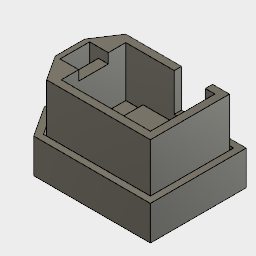
trrs-wssm-housing (Autodesk Fusion 360 design; units mm, degrees)
Autodesk Fusion 360 part; units mm, degrees
sketch "Sketch1" plane through (0, 0, 0) normal (0, 1, 0) x (1, 0, 0)
  line L0 (10.55, -8.05) -> (-10.55, -8.05)
  line L1 (-10.55, -8.05) -> (-10.55, 8.05)
  line L2 (-10.55, 8.05) -> (10.55, 8.05)
  line L3 (10.55, 8.05) -> (10.55, -8.05)
  line L4 (10.55, -8.05) -> (-10.55, 8.05) construction
  line L5 (-10.55, -8.05) -> (10.55, 8.05) construction
  dimension "d1" = 21.1
  dimension "d2" = 16.1
  measures "d1" distance of L1.end L2.end
  measures "d2" distance of L0.end L1.end
extrude "Extrude1" add sketch "Sketch1" along normal blind 3.5 makes body 1
sketch "Sketch2" plane through (0, 3.5, 0) normal (0, 1, 0) x (-1, 0, 0)
  line L0 (-10.55, -8.05) -> (10.55, -8.05)
  line L1 (10.55, -8.05) -> (10.55, 8.05)
  line L2 (10.55, 8.05) -> (-10.55, 8.05)
  line L3 (-10.55, 8.05) -> (-10.55, -8.05)
  line L4 (-9.05, 6.55) -> (9.05, 6.55)
  line L5 (9.05, 6.55) -> (9.05, -6.55)
  line L6 (9.05, -6.55) -> (-9.05, -6.55)
  line L7 (-9.05, -6.55) -> (-9.05, 6.55)
  line L8 (-9.05, 6.55) -> (9.05, -6.55) construction
  line L9 (9.05, 6.55) -> (-9.05, -6.55) construction
  dimension "d5" = 18.1
  dimension "d6" = 13.1
  measures "d5" distance of L5.end L6.end
  measures "d6" distance of L4.end L5.end
extrude "Extrude2" cut sketch "Sketch2" against normal blind 1.5 contours L4 L5 L6 L7 bodies 1
extrude "Extrude3" add 1 faces at (-3.0167, 3.5, -7.55) along direction (0, 1, 0) blind 5.7 on bodies 1 bodies 1
sketch "Sketch3" plane through (0, 9.2, 0) normal (0, 1, 0) x (-1, 0, 0)
  line L0 (9.05, 6.55) -> (9.05, -6.55)
  line L1 (9.05, -6.55) -> (-9.05, -6.55)
  line L2 (-9.05, -6.55) -> (-9.05, 6.55)
  line L3 (-9.05, 6.55) -> (9.05, 6.55)
  line L4 (-10.55, -8.05) -> (10.55, -8.05)
  line L5 (10.55, -8.05) -> (10.55, 8.05)
  line L6 (10.55, 8.05) -> (-10.55, 8.05)
  line L7 (-10.55, 8.05) -> (-10.55, -8.05)
  line L8 (-9.05, -6.55) -> (-7.1, -6.55)
  line L9 (-7.1, -6.55) -> (-7.1, -8.05)
  line L10 (-7.1, -8.05) -> (-9.05, -8.05)
  line L11 (-9.05, -8.05) -> (-9.05, -6.55)
  line L12 (-7.1, -6.55) -> (-0.8, -6.55)
  line L13 (-0.8, -6.55) -> (-0.8, -8.05)
  line L14 (-0.8, -8.05) -> (-7.1, -8.05)
  line L15 (-7.1, -8.05) -> (-7.1, -6.55)
  dimension "d11" = 1.95
  dimension "d12" = 6.3
  measures "d11" distance of L1.end L8.end
  measures "d12" distance of L8.end L12.end
extrude "Extrude4" cut sketch "Sketch3" against normal blind 5.7 contours L1 L4 L9 L12 L13 L14 L15 bodies 1
sketch "Sketch4" plane through (0, 2, 0) normal (0, 1, 0) x (-1, 0, 0)
  line L0 (-9.05, -6.55) -> (9.05, -6.55)
  line L1 (9.05, -6.55) -> (9.05, 6.55)
  line L2 (9.05, 6.55) -> (-9.05, 6.55)
  line L3 (-9.05, 6.55) -> (-9.05, -6.55)
  line L4 (-0.8, -6.55) -> (-7.1, -6.55)
  line L5 (-7.1, -6.55) -> (-7.1, -8.05)
  line L6 (-7.1, -8.05) -> (-0.8, -8.05)
  line L7 (-0.8, -8.05) -> (-0.8, -6.55)
  line L8 (9.05, -6.55) -> (5.55, -6.55)
  line L9 (5.55, -6.55) -> (5.55, 6.55)
  line L10 (5.55, 6.55) -> (9.05, 6.55)
  line L11 (9.05, 6.55) -> (9.05, -6.55)
  dimension "d15" = 3.5
  measures "d15" distance of L0.end L8.end
extrude "Extrude5" cut sketch "Sketch4" against normal blind 1 contours L0 L1 L2 L8 L9 L10 L11 bodies 1
sketch "Sketch5" plane through (0, 9.2, 0) normal (0, 1, 0) x (-1, 0, 0)
  line L0 (-7.1, -8.05) -> (-7.1, -6.55)
  line L1 (-7.1, -6.55) -> (-9.05, -6.55)
  line L2 (-9.05, -6.55) -> (-9.05, 6.55)
  line L3 (-9.05, 6.55) -> (9.05, 6.55)
  line L4 (9.05, 6.55) -> (9.05, -6.55)
  line L5 (9.05, -6.55) -> (-0.8, -6.55)
  line L6 (-0.8, -6.55) -> (-0.8, -8.05)
  line L7 (-0.8, -8.05) -> (10.55, -8.05)
  line L8 (10.55, -8.05) -> (10.55, 8.05)
  line L9 (10.55, 8.05) -> (-10.55, 8.05)
  line L10 (-10.55, 8.05) -> (-10.55, -8.05)
  line L11 (-10.55, -8.05) -> (-7.1, -8.05)
  line L12 (12.85, -3) -> (8.25, -3)
  line L13 (8.25, -3) -> (8.25, 3)
  line L14 (8.25, 3) -> (12.85, 3)
  line L15 (12.85, 3) -> (12.85, -3)
  line L16 (12.85, -3) -> (8.25, 3) construction
  line L17 (8.25, -3) -> (12.85, 3) construction
  line L18 (12.85, -3) -> (13.85, -3)
  line L19 (13.85, -3) -> (13.85, 3)
  line L20 (13.85, 3) -> (12.85, 3)
  line L21 (12.85, 3) -> (12.85, -3)
  line L22 (10.55, -8.05) -> (10.55, 8.05)
  line L23 (10.55, 8.05) -> (13.85, 3)
  line L24 (13.85, -3) -> (10.55, -8.05)
  point P0 (10.55, 0)
  dimension "d18" = 4.6
  dimension "d19" = 6
  dimension "d20" = 1
  measures "d18" distance of L13.end L14.end
  measures "d19" distance of L12.end L13.end
  measures "d20" distance of L12.start L18.end
extrude "Extrude6" add sketch "Sketch5" against normal blind 9.2 contours L8 L14 L20 L22 L23 | L8 L12 L14 L15 L21 L22 | L15 L18 L19 L20 L21 | L8 L12 L18 L22 L24 bodies 1
sketch "Sketch6" plane through (0, 9.2, 0) normal (0, 1, 0) x (-1, 0, 0)
  line L0 (-7.1, -8.05) -> (-7.1, -6.55)
  line L1 (-7.1, -6.55) -> (-9.05, -6.55)
  line L2 (-9.05, -6.55) -> (-9.05, 6.55)
  line L3 (-9.05, 6.55) -> (9.05, 6.55)
  line L4 (9.05, 6.55) -> (9.05, -6.55)
  line L5 (9.05, -6.55) -> (-0.8, -6.55)
  line L6 (-0.8, -6.55) -> (-0.8, -8.05)
  line L7 (-0.8, -8.05) -> (10.55, -8.05)
  line L8 (10.55, -8.05) -> (13.85, -3)
  line L9 (13.85, -3) -> (13.85, 3)
  line L10 (13.85, 3) -> (10.55, 8.05)
  line L11 (10.55, 8.05) -> (-10.55, 8.05)
  line L12 (-10.55, 8.05) -> (-10.55, -8.05)
  line L13 (-10.55, -8.05) -> (-7.1, -8.05)
  line L14 (13.85, -3) -> (12.85, -3)
  line L15 (12.85, -3) -> (12.85, 3)
  line L16 (12.85, 3) -> (13.85, 3)
  line L17 (13.85, 3) -> (13.85, -3)
  line L18 (12.85, -3) -> (11.05, -3)
  line L19 (11.05, -3) -> (11.05, 3)
  line L20 (11.05, 3) -> (12.85, 3)
  line L21 (12.85, 3) -> (12.85, -3)
  dimension "d23" = 1
  dimension "d24" = 1.8
  measures "d23" distance of L8.end L14.end
  measures "d24" distance of L14.end L18.end
extrude "Extrude7" cut sketch "Sketch6" against normal blind 7.2 contours L15 L18 L19 L20 L21 bodies 1
extrude "Extrude8" add 1 faces at (-9.7167, 9.2, -1) along direction (0, 1, 0) blind 2 on bodies 1 bodies 1
sketch "Sketch7" plane through (0, 11.2, 0) normal (0, 1, 0) x (-1, 0, 0)
  line L0 (11.05, -3) -> (11.05, 3)
  line L1 (11.05, 3) -> (12.85, 3)
  line L2 (12.85, 3) -> (12.85, -3)
  line L3 (12.85, -3) -> (11.05, -3)
  line L4 (-7.1, -8.05) -> (-7.1, -6.55)
  line L5 (-7.1, -6.55) -> (-9.05, -6.55)
  line L6 (-9.05, -6.55) -> (-9.05, 6.55)
  line L7 (-9.05, 6.55) -> (9.05, 6.55)
  line L8 (9.05, 6.55) -> (9.05, -6.55)
  line L9 (9.05, -6.55) -> (-0.8, -6.55)
  line L10 (-0.8, -6.55) -> (-0.8, -8.05)
  line L11 (-0.8, -8.05) -> (10.55, -8.05)
  line L12 (10.55, -8.05) -> (13.85, -3)
  line L13 (13.85, -3) -> (13.85, 3)
  line L14 (13.85, 3) -> (10.55, 8.05)
  line L15 (10.55, 8.05) -> (-10.55, 8.05)
  line L16 (-10.55, 8.05) -> (-10.55, -8.05)
  line L17 (-10.55, -8.05) -> (-7.1, -8.05)
  line L18 (11.05, -3) -> (9.05, -3)
  line L19 (9.05, -3) -> (9.05, 3)
  line L20 (9.05, 3) -> (11.05, 3)
  line L21 (11.05, 3) -> (11.05, -3)
extrude "Extrude9" cut sketch "Sketch7" against normal blind 2 contours L0 L8 L18 L19 L20 L21 bodies 1
copy_body "Body->Comp1" bodies 1 removing the originals makes body 2 in component "WSSM-03: Lower Half "
sketch "Sketch1 (2)" plane through (0, 11.2, 0) normal (0, 1, 0) x (-1, 0, 0) in component "WSSM-04: Upper Half"
  line L0 (9.05, 3) -> (12.85, 3)
  line L1 (12.85, 3) -> (12.85, -3)
  line L2 (12.85, -3) -> (9.05, -3)
  line L3 (9.05, -3) -> (9.05, -6.55)
  line L4 (9.05, -6.55) -> (-0.8, -6.55)
  line L5 (-0.8, -6.55) -> (-0.8, -8.05)
  line L6 (-0.8, -8.05) -> (10.55, -8.05)
  line L7 (10.55, -8.05) -> (13.85, -3)
  line L8 (13.85, -3) -> (13.85, 3)
  line L9 (13.85, 3) -> (10.55, 8.05)
  line L10 (10.55, 8.05) -> (-10.55, 8.05)
  line L11 (-10.55, 8.05) -> (-10.55, -8.05)
  line L12 (-10.55, -8.05) -> (-7.1, -8.05)
  line L13 (-7.1, -8.05) -> (-7.1, -6.55)
  line L14 (-7.1, -6.55) -> (-9.05, -6.55)
  line L15 (-9.05, -6.55) -> (-9.05, 6.55)
  line L16 (-9.05, 6.55) -> (9.05, 6.55)
  line L17 (9.05, 6.55) -> (9.05, 3)
  line L18 (-9.05, 6.55) -> (-0.8, 6.55)
  line L19 (-0.8, 6.55) -> (-0.8, -6.55)
  line L20 (-0.8, -6.55) -> (-9.05, -6.55)
  line L21 (-9.05, -6.55) -> (-9.05, 6.55)
  line L22 (-0.8, -8.05) -> (-7.1, -8.05)
  line L23 (-7.1, -8.05) -> (-7.1, -6.55)
  line L24 (-7.1, -6.55) -> (-0.8, -6.55)
  line L25 (-0.8, -6.55) -> (-0.8, -8.05)
extrude "Extrude1'" add sketch "Sketch1 (2)" against normal blind 1.85 separate body contours L14 L15 L16 L18 L19 L20 L21 L24 | L5 L13 L20 L22 L23 L24 L25 makes body 3 in component "WSSM-04: Upper Half"
move_face "OffsetFaces1" offset -0.09 1 faces at (9.05, 10.5833, -2.1833) on bodies 3 in component "WSSM-04: Upper Half"
move_face "OffsetFaces2" offset -0.09 1 faces at (3.52, 9.9667, 6.55) on bodies 3 in component "WSSM-04: Upper Half"
move_face "OffsetFaces3" offset -0.09 1 faces at (7.72, 10.5833, -6.55) on bodies 3 in component "WSSM-04: Upper Half"
move_face "OffsetFaces4" offset -0.15 1 faces at (7.1, 10.5833, -7.52) on bodies 3 in component "WSSM-04: Upper Half"
sketch "Sketch2 (2)" plane through (0, 11.2, 0) normal (0, 1, 0) x (-1, 0, 0) in component "WSSM-04: Upper Half"
  line L0 (9.05, 3) -> (12.85, 3)
  line L1 (12.85, 3) -> (12.85, -3)
  line L2 (12.85, -3) -> (9.05, -3)
  line L3 (9.05, -3) -> (9.05, -6.55)
  line L4 (9.05, -6.55) -> (-0.8, -6.55)
  line L5 (-0.8, -6.55) -> (-0.8, -8.05)
  line L6 (-0.8, -8.05) -> (10.55, -8.05)
  line L7 (10.55, -8.05) -> (13.85, -3)
  line L8 (13.85, -3) -> (13.85, 3)
  line L9 (13.85, 3) -> (10.55, 8.05)
  line L10 (10.55, 8.05) -> (-10.55, 8.05)
  line L11 (-10.55, 8.05) -> (-10.55, -8.05)
  line L12 (-10.55, -8.05) -> (-7.1, -8.05)
  line L13 (-7.1, -8.05) -> (-7.1, -6.55)
  line L14 (-7.1, -6.55) -> (-9.05, -6.55)
  line L15 (-9.05, -6.55) -> (-9.05, 6.55)
  line L16 (-9.05, 6.55) -> (9.05, 6.55)
  line L17 (9.05, 6.55) -> (9.05, 3)
  line L18 (9.05, -6.55) -> (-0.8, -6.55)
  line L19 (-0.8, -6.55) -> (-0.8, 6.46)
  line L20 (-0.8, 6.46) -> (9.05, 6.46)
  line L21 (9.05, 6.46) -> (9.05, -6.55)
  line L22 (9.05, -3) -> (12.85, -3)
  line L23 (12.85, -3) -> (12.85, 3)
  line L24 (12.85, 3) -> (9.05, 3)
  line L25 (9.05, 3) -> (9.05, -3)
  point P0 (-0.8, 6.46)
extrude "Extrude2'" add sketch "Sketch2 (2)" against normal blind 1 contours L3 L4 L17 L18 L19 L20 L21 L25 | L0 L1 L2 L21 L22 L23 L24 L25 bodies 3 in component "WSSM-04: Upper Half"
move_face "OffsetFaces5" offset -0.15 1 faces at (-9.05, 10.8667, 5.3067) on bodies 3 in component "WSSM-04: Upper Half"
move_face "OffsetFaces6" offset -0.09 1 faces at (-10.2167, 10.8667, 3) on bodies 3 in component "WSSM-04: Upper Half"
move_face "OffsetFaces7" offset -0.15 1 faces at (-12.85, 10.8667, 0.94) on bodies 3 in component "WSSM-04: Upper Half"
move_face "OffsetFaces8" offset -0.09 1 faces at (-11.4833, 10.8667, -3) on bodies 3 in component "WSSM-04: Upper Half"
move_face "OffsetFaces9" offset -0.15 1 faces at (-9.05, 10.8667, -4.1233) on bodies 3 in component "WSSM-04: Upper Half"
move_face "OffsetFaces10" offset -0.09 1 faces at (-5.6667, 10.5333, -6.55) on bodies 3 in component "WSSM-04: Upper Half"
move_face "OffsetFaces11" offset -0.09 1 faces at (0.8, 10.25, -7.52) on bodies 3 in component "WSSM-04: Upper Half"
sketch "Sketch3 (2)" plane through (0, 11.2, 0) normal (0, 1, 0) x (-1, 0, 0) in component "WSSM-04: Upper Half"
  line L0 (9.05, 3) -> (12.85, 3)
  line L1 (12.85, 3) -> (12.85, -3)
  line L2 (12.85, -3) -> (9.05, -3)
  line L3 (9.05, -3) -> (9.05, -6.55)
  line L4 (9.05, -6.55) -> (-0.8, -6.55)
  line L5 (-0.8, -6.55) -> (-0.8, -8.05)
  line L6 (-0.8, -8.05) -> (10.55, -8.05)
  line L7 (10.55, -8.05) -> (13.85, -3)
  line L8 (13.85, -3) -> (13.85, 3)
  line L9 (13.85, 3) -> (10.55, 8.05)
  line L10 (10.55, 8.05) -> (-10.55, 8.05)
  line L11 (-10.55, 8.05) -> (-10.55, -8.05)
  line L12 (-10.55, -8.05) -> (-7.1, -8.05)
  line L13 (-7.1, -8.05) -> (-7.1, -6.55)
  line L14 (-7.1, -6.55) -> (-9.05, -6.55)
  line L15 (-9.05, -6.55) -> (-9.05, 6.55)
  line L16 (-9.05, 6.55) -> (9.05, 6.55)
  line L17 (9.05, 6.55) -> (9.05, 3)
  line L18 (-10.55, -8.05) -> (10.55, -8.05)
  line L19 (13.85, -3) -> (13.85, 3)
  line L20 (10.55, 8.05) -> (-10.55, 8.05)
extrude "Extrude3'" add sketch "Sketch3 (2)" along normal blind 2 bodies 3 in component "WSSM-04: Upper Half"
sketch "Sketch4 (2)" plane through (-13.85, 0, 0) normal (-1, 0, 0) x (0, 0, 1) in component "WSSM-04: Upper Half"
  line L0 (-3, 11.2) -> (3, 11.2)
  line L1 (3, 11.2) -> (3, 13.2)
  line L2 (3, 13.2) -> (-3, 13.2)
  line L3 (-3, 13.2) -> (-3, 11.2)
  line L4 (-3, 11.2) -> (3, 11.2)
  line L5 (3, 11.2) -> (3, 12.2)
  line L6 (3, 12.2) -> (-3, 12.2)
  line L7 (-3, 12.2) -> (-3, 11.2)
extrude "Extrude4'" cut sketch "Sketch4 (2)" against normal blind 1 contours L0 L1 L3 L4 L5 L6 L7 bodies 3 in component "WSSM-04: Upper Half"
sketch "Sketch5 (2)" plane through (10.55, 0, 0) normal (1, 0, 0) x (0, 0, -1) in component "WSSM-04: Upper Half"
  line L0 (-8.05, 11.2) -> (8.05, 11.2)
  line L1 (8.05, 11.2) -> (8.05, 13.2)
  line L2 (8.05, 13.2) -> (-8.05, 13.2)
  line L3 (-8.05, 13.2) -> (-8.05, 11.2)
  line L4 (3, 12.2) -> (-3, 12.2)
  line L5 (-3, 12.2) -> (-3, 10.2)
  line L6 (-3, 10.2) -> (3, 10.2)
  line L7 (3, 10.2) -> (3, 12.2)
  line L8 (3, 12.2) -> (-3, 10.2) construction
  line L9 (-3, 12.2) -> (3, 10.2) construction
  line L10 (-3, 12.2) -> (3, 12.2)
  line L11 (3, 12.2) -> (3, 11.2)
  line L12 (3, 11.2) -> (-3, 11.2)
  line L13 (-3, 11.2) -> (-3, 12.2)
  point P0 (0, 11.2)
  dimension "d50" = 6
  dimension "d51" = 2
  dimension "d52" = 6
  dimension "d53" = 1
  measures "d50" distance of L5.end L6.end
  measures "d51" distance of L4.end L5.end
  measures "d52" distance of L4.end L4.start
  measures "d53" distance of L4.end L12.end
extrude "Extrude5'" cut sketch "Sketch5 (2)" against normal blind 1 contours L0 L4 L5 L7 L10 L11 L12 L13 bodies 3 in component "WSSM-04: Upper Half"
sketch "Sketch8" plane through (0, 10.2, 0) normal (0, -1, 0) x (1, 0, 0)
  line L0 (-12.7, -2.91) -> (-8.9, -2.91)
  line L1 (-8.9, -2.91) -> (-8.9, -6.46)
  line L2 (-8.9, -6.46) -> (0.89, -6.46)
  line L3 (0.89, -6.46) -> (0.89, 6.46)
  line L4 (0.89, 6.46) -> (-8.9, 6.46)
  line L5 (-8.9, 6.46) -> (-8.9, 2.91)
  line L6 (-8.9, 2.91) -> (-12.7, 2.91)
  line L7 (-12.7, 2.91) -> (-12.7, -2.91)
  line L8 (-8.9, 6.46) -> (0.89, 6.46)
  line L9 (0.89, 6.46) -> (0.89, -6.46)
  line L10 (0.89, -6.46) -> (-8.9, -6.46)
  line L11 (-8.9, -6.46) -> (-8.9, 6.46)
extrude "Extrude6'" add sketch "Sketch8" along normal up to surface (0.85 mm away) contours L1 L2 L3 L4 L5 L8 L9 L10 L11 bodies 3 in component "WSSM-04: Upper Half"
sketch "Sketch9" plane through (-13.85, 0, 0) normal (-1, 0, 0) x (0, 0, 1)
  line L0 (-3, 11.2) -> (-3, 0)
  line L1 (-3, 0) -> (3, 0)
  line L2 (3, 0) -> (3, 11.2)
  line L3 (3, 11.2) -> (-3, 11.2)
  line L4 (1.75, 6.6) -> (-1.75, 6.6)
  line L5 (-1.75, 6.6) -> (-1.75, 4.6)
  line L6 (-1.75, 4.6) -> (1.75, 4.6)
  line L7 (1.75, 4.6) -> (1.75, 6.6)
  line L8 (1.75, 6.6) -> (-1.75, 4.6) construction
  line L9 (-1.75, 6.6) -> (1.75, 4.6) construction
  point P0 (0, 5.6)
  dimension "d58" = 3.5
  dimension "d59" = 2
  measures "d58" distance of L5.end L6.end
  measures "d59" distance of L4.end L5.end
extrude "Extrude1''" add sketch "Sketch9" along normal blind 2.5 contours L4 L5 L6 L7 bodies 2 in component "WSSM-03: Lower Half "
fillet "Fillet1" radius 0.2 4 edges at (-13.85, 6.6, 0) (-13.85, 5.6, -1.75) (-13.85, 4.6, 0) (-13.85, 5.6, 1.75) on bodies 2 in component "WSSM-03: Lower Half "
fillet "Fillet2" radius 0.2 8 edges at (-13.9086, 6.6586, -1.8086) (-15.2, 6.6, -1.75) (-13.9086, 6.6586, 1.8086) (-15.2, 6.6, 1.75) (-13.9086, 4.5414, -1.8086) (-15.2, 4.6, -1.75) (-13.9086, 4.5414, 1.8086) (-15.2, 4.6, 1.75) on bodies 2 in component "WSSM-03: Lower Half "
fillet "Fillet3" radius 0.2 8 edges at (-16.35, 6.5414, -1.6914) (-16.35, 5.6, -1.75) (-16.35, 4.6586, -1.6914) (-16.35, 4.6, 0) (-16.35, 4.6586, 1.6914) (-16.35, 5.6, 1.75) (-16.35, 6.5414, 1.6914) (-16.35, 6.6, 0) on bodies 2 in component "WSSM-03: Lower Half "
extrude "Extrude2''" add 1 faces at (3.5167, 0, 2.6833) along direction (0, -1, 0) blind 1.3 on bodies 2 bodies 2 in component "WSSM-03: Lower Half "
sketch "Sketch10" plane through (0, -1.3, 0) normal (0, -1, 0) x (1, 0, 0)
  line L0 (-10.55, -8.05) -> (10.55, -8.05)
  line L1 (10.55, -8.05) -> (10.55, 8.05)
  line L2 (10.55, 8.05) -> (-10.55, 8.05)
  line L3 (-10.55, 8.05) -> (-13.85, 3)
  line L4 (-13.85, 3) -> (-13.85, -3)
  line L5 (-13.85, -3) -> (-10.55, -8.05)
  line L6 (-15.55, 3.5062) -> (-15.55, -3.5062)
  line L7 (-15.55, -3.5062) -> (-11.4699, -9.75)
  line L8 (-11.4699, -9.75) -> (12.25, -9.75)
  line L9 (12.25, -9.75) -> (12.25, 9.75)
  line L10 (12.25, 9.75) -> (-11.4699, 9.75)
  line L11 (-11.4699, 9.75) -> (-15.55, 3.5062)
  dimension "d67" = 1.7
extrude "Extrude1'''" add sketch "Sketch10" along normal blind 4 separate body contours L0 L1 L2 L3 L4 L5 | L6 L7 L8 L9 L10 L11 makes body 4 in component "TestStand Mount"
sketch "Sketch1 (3)" plane through (0, -1.3, 0) normal (0, 1, 0) x (-1, 0, 0) in component "TestStand Mount"
  line L0 (15.55, 3.5062) -> (11.4699, 9.75)
  line L1 (11.4699, 9.75) -> (-12.25, 9.75)
  line L2 (-12.25, 9.75) -> (-12.25, -9.75)
  line L3 (-12.25, -9.75) -> (11.4699, -9.75)
  line L4 (11.4699, -9.75) -> (15.55, -3.5062)
  line L5 (15.55, -3.5062) -> (15.55, 3.5062)
  line L6 (-10.95, -8.45) -> (10.7664, -8.45)
  line L7 (10.7664, -8.45) -> (14.25, -3.1191)
  line L8 (14.25, -3.1191) -> (14.25, 3.1191)
  line L9 (14.25, 3.1191) -> (10.7664, 8.45)
  line L10 (10.7664, 8.45) -> (-10.95, 8.45)
  line L11 (-10.95, 8.45) -> (-10.95, -8.45)
  dimension "d70" = 1.3
extrude "Extrude2'''" add sketch "Sketch1 (3)" along normal blind 3 bodies 4 in component "TestStand Mount"
component "WSSM-03: Lower Half " placed x (1, 0, 0) y (0, 1, 0) z (0, 0, 1) at (0, 0, 0)
component "WSSM-04: Upper Half" placed x (1, 0, 0) y (0, 1, 0) z (0, 0, 1) at (0, 0, 0)
component "TestStand Mount" placed x (1, 0, 0) y (0, 1, 0) z (0, 0, 1) at (0, 0, 0)
equation "clearance = -0.09 mm"
equation "d34 = clearance"
equation "d35 = clearance"
equation "d40 = clearance"
equation "d42 = clearance"
equation "d44 = clearance"
equation "d45 = clearance"
